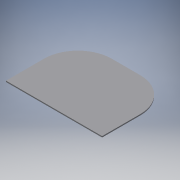
# Autodesk Inventor part: BottleHolderCap
Saved by Autodesk Inventor 2017 (Build 210142000, 142)
## iProperties
Created: 2016-11-04
Part Number: BottleHolderCap
Material: Generic
Document SubType Name: Modeling
Designer: Camilo
Density: 1 g/cm^3
Appearance: Default
Author: Camilo
Autodesk Inventor part; units mm, degrees
ref_plane "YZ Plane" through (0, 0, 0) normal (1, 0, 0) x (0, 1, 0)
ref_plane "XZ Plane" through (0, 0, 0) normal (0, 1, 0) x (-1, 0, 0)
ref_plane "XY Plane" through (0, 0, 0) normal (0, 0, 1) x (1, 0, 0)
sketch "Sketch1" plane through (0, 0, 0) normal (0, 0, 1) x (1, 0, 0)
  line L0 (-73.25, -41.4701) -> (-73.25, 14.3616) construction
  arc A0 (-24.5816, 63.0299) -> (-73.25, 14.3616) centre (-24.5816, 14.3616) ccw construction
  line L1 (-24.5816, 63.0299) -> (24.5816, 63.0299) construction
  arc A1 (73.25, 14.3616) -> (24.5816, 63.0299) centre (24.5816, 14.3616) ccw construction
  line L2 (73.25, 14.3616) -> (73.25, -41.4701) construction
  line L3 (73.25, -41.4701) -> (-73.25, -41.4701) construction
  line L4 (-80.75, -48.9701) -> (80.75, -48.9701) construction
  line L5 (80.75, -48.9701) -> (80.75, 14.3616) construction
  arc A2 (80.75, 14.3616) -> (24.5816, 70.5299) centre (24.5816, 14.3616) ccw construction
  line L6 (24.5816, 70.5299) -> (-24.5816, 70.5299) construction
  arc A3 (-24.5816, 70.5299) -> (-80.75, 14.3616) centre (-24.5816, 14.3616) ccw construction
  line L7 (-80.75, 14.3616) -> (-80.75, -48.9701) construction
  arc A4 (83.25, 14.3616) -> (24.5816, 73.0299) centre (24.5816, 14.3616) ccw
  line L8 (83.25, 14.3616) -> (83.25, -51.4701)
  line L9 (83.25, -51.4701) -> (-83.25, -51.4701)
  line L10 (-83.25, -51.4701) -> (-83.25, 14.3616)
  arc A5 (-24.5816, 73.0299) -> (-83.25, 14.3616) centre (-24.5816, 14.3616) ccw
  line L11 (-24.5816, 73.0299) -> (24.5816, 73.0299)
  point P0 (0, 0)
  dimension "d0" = 2.5
  constraints: 8 end point, 4 point on circle, 2 centre point, 5 other
  measures "d0" distance between parallel lines of L9 L4
extrude "Extrusion1" add sketch "Sketch1" along normal blind 2
sketch "Sketch2" plane through (0, 0, 0) normal (0, 0, -1) x (-1, 0, 0)
  line L0 (73.25, -41.4701) -> (73.25, 14.3616) construction
  arc A0 (73.25, 14.3616) -> (24.5816, 63.0299) centre (24.5816, 14.3616) ccw construction
  line L1 (24.5816, 63.0299) -> (-24.5816, 63.0299) construction
  arc A1 (-24.5816, 63.0299) -> (-73.25, 14.3616) centre (-24.5816, 14.3616) ccw construction
  line L2 (-73.25, 14.3616) -> (-73.25, -41.4701) construction
  line L3 (-73.25, -41.4701) -> (73.25, -41.4701) construction
  line L4 (80.75, -48.9701) -> (-80.75, -48.9701) construction
  line L5 (-80.75, -48.9701) -> (-80.75, 14.3616) construction
  arc A2 (-24.5816, 70.5299) -> (-80.75, 14.3616) centre (-24.5816, 14.3616) ccw construction
  line L6 (-24.5816, 70.5299) -> (24.5816, 70.5299) construction
  arc A3 (80.75, 14.3616) -> (24.5816, 70.5299) centre (24.5816, 14.3616) ccw construction
  line L7 (80.75, 14.3616) -> (80.75, -48.9701) construction
  line L8 (-73.1, -41.3201) -> (-73.1, 14.3616)
  arc A4 (-24.5816, 62.8799) -> (-73.1, 14.3616) centre (-24.5816, 14.3616) ccw
  line L9 (-24.5816, 62.8799) -> (24.5816, 62.8799)
  arc A5 (73.1, 14.3616) -> (24.5816, 62.8799) centre (24.5816, 14.3616) ccw
  line L10 (73.1, 14.3616) -> (73.1, -41.3201)
  line L11 (73.1, -41.3201) -> (-73.1, -41.3201)
  line L12 (-71.6, 14.3616) -> (-71.6, -39.8201)
  line L13 (-71.6, -39.8201) -> (71.6, -39.8201)
  line L14 (71.6, -39.8201) -> (71.6, 14.3616)
  arc A6 (71.6, 14.3616) -> (24.5816, 61.3799) centre (24.5816, 14.3616) ccw
  line L15 (24.5816, 61.3799) -> (-24.5816, 61.3799)
  arc A7 (-24.5816, 61.3799) -> (-71.6, 14.3616) centre (-24.5816, 14.3616) ccw
  point P0 (0, 0)
  dimension "d3" = 0.15
  dimension "d4" = 1.5
  constraints: 16 end point, 8 point on circle, 4 centre point, 10 other
  measures "d3" distance between parallel lines of L3 L11
  measures "d4" distance between parallel lines of L11 L13
extrude "Extrusion2" add sketch "Sketch2" along normal blind 5
body "Solid1"
